Autodesk Fusion 360 part; units mm, degrees
(part 4 of 4)
component "Component'''''''''''''''''''''''''''''''''''''''''''''''''''''''''''''''''" placed x (1, 0, 0) y (0, 0, -1) z (0, 1, 0) at (-652.0041, 0, 260.2242)
component "Component''''''''''''''''''''''''''''''''''''''''''''''''''''''''''''''''''" placed x (1, 0, 0) y (0, 0, -1) z (0, 1, 0) at (-887.754, 0, 434.1846)
component "Component'''''''''''''''''''''''''''''''''''''''''''''''''''''''''''''''''''" placed x (1, 0, 0) y (0, 0, -1) z (0, 1, 0) at (-760.2499, 0, 618.8245)
component "Component''''''''''''''''''''''''''''''''''''''''''''''''''''''''''''''''''''" placed x (-1, 0, 0) y (0, 0, 1) z (0, 1, 0) at (1329.7999, 0, 193.6744)
component "Component'''''''''''''''''''''''''''''''''''''''''''''''''''''''''''''''''''''" placed x (1, 0, 0) y (0, 0, -1) z (0, 1, 0) at (-651.6501, 0, 768.8245)
component "Component''''''''''''''''''''''''''''''''''''''''''''''''''''''''''''''''''''''" placed x (1, 0, 0) y (0, 0, -1) z (0, 1, 0) at (-927.004, 0, 312.3743)
component "Component'''''''''''''''''''''''''''''''''''''''''''''''''''''''''''''''''''''''" placed x (1, 0, 0) y (0, 0, -1) z (0, 1, 0) at (-1162.7539, 0, 486.3346)
component "Component''''''''''''''''''''''''''''''''''''''''''''''''''''''''''''''''''''''''" placed x (1, 0, 0) y (0, 0, -1) z (0, 1, 0) at (-1008.1, 0, 618.8245)
component "Component'''''''''''''''''''''''''''''''''''''''''''''''''''''''''''''''''''''''''" placed x (1, 0, 0) y (0, 0, -1) z (0, 1, 0) at (-953.8001, 0, 693.8245)
component "Component''''''''''''''''''''''''''''''''''''''''''''''''''''''''''''''''''''''''''" placed x (0, 0, -1) y (-1, 0, 0) z (0, 1, 0) at (459.45, 0, 1770.9738)
component "Envelope1(Qty: 1)" placed x (0, 0, 1) y (1, 0, 0) z (0, 1, 0) at (0, 0, 0) in component "Arrange1"
equation "Thickness = 3.35 mm"
equation "Length = 50 mm"
equation "Width = 50 mm"
equation "Depth_of_slot = 10 mm"
equation "d5 = Thickness - Kerf - Clearance"
equation "d8 = Depth_of_slot + Kerf"
equation "d9 = Hexagon_side + Kerf"
equation "d10 = Width + Kerf"
equation "Width_of_small_Piece = 25 mm"
equation "d12 = Width_of_small_Piece + Kerf"
equation "d13 = Length + Kerf"
equation "Kerf = 0.15 mm"
equation "Hexagon_side = 30 mm"
equation "d20 = Length + Kerf"
equation "Clearance = 0.1 mm"
